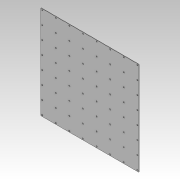
# Autodesk Inventor part: NozzleAligner
Saved by Autodesk Inventor 2020 (Build 240168000, 168)
## iProperties
Created: 2021-09-12
Part Number: NozzleAligner
Material: Generic
Document SubType Name: Modeling
Designer: DDeGo
Density: 1 g/cm^3
Appearance: Default
Author: DDeGo
Autodesk Inventor part; units mm, degrees
ref_plane "YZ Plane" through (0, 0, 0) normal (1, 0, 0) x (0, 1, 0)
ref_plane "XZ Plane" through (0, 0, 0) normal (0, 1, 0) x (-1, 0, 0)
ref_plane "XY Plane" through (0, 0, 0) normal (0, 0, 1) x (1, 0, 0)
sketch "Sketch1" plane through (0, 0, 0) normal (0, 0, 1) x (1, 0, 0)
  line L0 (-79, -75.5) -> (79, -75.5)
  line L1 (79, -75.5) -> (79, 75.5)
  line L2 (79, 75.5) -> (-79, 75.5)
  line L3 (-79, 75.5) -> (-79, -75.5)
  line L4 (-79, -75.5) -> (79, 75.5) construction
  line L5 (79, -75.5) -> (-79, 75.5) construction
  circle A0 centre (-77, -73.5) radius 1
  circle A1 centre (-55, -73.5) radius 1
  circle A2 centre (-33, -73.5) radius 1
  circle A3 centre (-11, -73.5) radius 1
  circle A4 centre (11, -73.5) radius 1
  circle A5 centre (33, -73.5) radius 1
  circle A6 centre (55, -73.5) radius 1
  circle A7 centre (77, -73.5) radius 1
  circle A8 centre (-77, -52.5) radius 1
  circle A9 centre (-55, -52.5) radius 1
  circle A10 centre (-33, -52.5) radius 1
  circle A11 centre (-11, -52.5) radius 1
  circle A12 centre (11, -52.5) radius 1
  circle A13 centre (33, -52.5) radius 1
  circle A14 centre (55, -52.5) radius 1
  circle A15 centre (77, -52.5) radius 1
  circle A16 centre (-77, -31.5) radius 1
  circle A17 centre (-55, -31.5) radius 1
  circle A18 centre (-33, -31.5) radius 1
  circle A19 centre (-11, -31.5) radius 1
  circle A20 centre (11, -31.5) radius 1
  circle A21 centre (33, -31.5) radius 1
  circle A22 centre (55, -31.5) radius 1
  circle A23 centre (77, -31.5) radius 1
  circle A24 centre (-77, -10.5) radius 1
  circle A25 centre (-55, -10.5) radius 1
  circle A26 centre (-33, -10.5) radius 1
  circle A27 centre (-11, -10.5) radius 1
  circle A28 centre (11, -10.5) radius 1
  circle A29 centre (33, -10.5) radius 1
  circle A30 centre (55, -10.5) radius 1
  circle A31 centre (77, -10.5) radius 1
  circle A32 centre (-77, 10.5) radius 1
  circle A33 centre (-55, 10.5) radius 1
  circle A34 centre (-33, 10.5) radius 1
  circle A35 centre (-11, 10.5) radius 1
  circle A36 centre (11, 10.5) radius 1
  circle A37 centre (33, 10.5) radius 1
  circle A38 centre (55, 10.5) radius 1
  circle A39 centre (77, 10.5) radius 1
  circle A40 centre (-77, 31.5) radius 1
  circle A41 centre (-55, 31.5) radius 1
  circle A42 centre (-33, 31.5) radius 1
  circle A43 centre (-11, 31.5) radius 1
  circle A44 centre (11, 31.5) radius 1
  circle A45 centre (33, 31.5) radius 1
  circle A46 centre (55, 31.5) radius 1
  circle A47 centre (77, 31.5) radius 1
  circle A48 centre (-77, 52.5) radius 1
  circle A49 centre (-55, 52.5) radius 1
  circle A50 centre (-33, 52.5) radius 1
  circle A51 centre (-11, 52.5) radius 1
  circle A52 centre (11, 52.5) radius 1
  circle A53 centre (33, 52.5) radius 1
  circle A54 centre (55, 52.5) radius 1
  circle A55 centre (77, 52.5) radius 1
  circle A56 centre (-77, 73.5) radius 1
  circle A57 centre (-55, 73.5) radius 1
  circle A58 centre (-33, 73.5) radius 1
  circle A59 centre (-11, 73.5) radius 1
  circle A60 centre (11, 73.5) radius 1
  circle A61 centre (33, 73.5) radius 1
  circle A62 centre (55, 73.5) radius 1
  circle A63 centre (77, 73.5) radius 1
  point P0 (0, 0)
  dimension "d0" = 2
  dimension "d3" = 22
  dimension "d6" = 21
  dimension "d9" = 2
  dimension "d10" = 2
  dimension "d11" = 2
  dimension "d12" = 2
  constraints: 64 centre point, 12 end point, 2 horizontal, 2 midpoint, 2 parallel, 1 perpendicular, 1 vertical, 126 other
  measures "d0" diameter of A0
  measures "d3" distance of A0.centre A1.centre
  measures "d6" distance of A0.centre A8.centre
  measures "d9" distance from line of L0 A0.centre
  measures "d10" distance from line of L3 A8.centre
  measures "d11" distance from line of L2 A56.centre
  measures "d12" distance from line of L1 A7.centre
extrude "Extrusion1" add sketch "Sketch1" along normal blind 0.6
body "Solid1"
